Autodesk Inventor part; units mm, degrees
(part 2 of 2)
sketch "Sketch8" plane through (0, 0, 3) normal (0, 0, 1) x (1, 0, 0)
  line L0 (210.1, -2) -> (210.1, -24.3525) projected
  line L1 (210.1, -2) -> (212.6, -2)
  line L2 (212.6, -2) -> (212.6, -5)
  line L3 (212.6, -5) -> (210.1, -5)
  line L4 (210.1, -5) -> (210.1, -2)
  point P0 (0, 0)
  dimension "d104" = 2.5
  dimension "d105" = 3
  constraints: 8 end point, 2 parallel, 1 horizontal, 1 perpendicular
  measures "d104" distance of L2.end L3.end
  measures "d105" distance of L1.end L2.end
extrude "Extrusion8" cut sketch "Sketch8" against normal blind 2
equation "\"d1\" = d0"
equation "\"d2\" = sw"
equation "\"d3\" = sw"
equation "\"d4\" = sw"
equation "\"d5\" = sw"
equation "\"d6\" = sw"
equation "\"d7\" = sw"
equation "\"d8\" = sw"
equation "\"d9\" = sw"
equation "\"d10\" = sw"
equation "\"d11\" = sw"
equation "\"d12\" = sw"
equation "\"d13\" = sw"
equation "\"d14\" = sw"
equation "\"d15\" = sw"
equation "\"d16\" = sw"
equation "\"d17\" = sw"
equation "\"d18\" = sw"
equation "\"d19\" = sw"
equation "\"d20\" = sw"
equation "\"d21\" = sw"
equation "\"d22\" = sw"
equation "\"d23\" = sw"
equation "\"d24\" = sw"
equation "\"d25\" = sw"
equation "\"d26\" = sw"
equation "\"d27\" = sw"
equation "\"d30\" = sw"
equation "\"d31\" = sw"
equation "\"d32\" = sw"
equation "\"d33\" = sw"
equation "\"d34\" = sw"
equation "\"d35\" = sw"
equation "\"d36\" = sw"
equation "\"d37\" = sw"
equation "\"d38\" = sw"
equation "\"d39\" = sw"
equation "\"d40\" = sw"
equation "\"d41\" = sw"
equation "\"d42\" = sw"
equation "\"d43\" = sw"
equation "\"d44\" = sw"
equation "\"d45\" = sw"
equation "\"d46\" = sw"
equation "\"d47\" = sw"
equation "\"d48\" = sw"
equation "\"d49\" = sw"
equation "\"d50\" = sw"
equation "\"d51\" = sw"
equation "\"d52\" = sw"
equation "\"d53\" = sw"
equation "\"d55\" = sw"
equation "\"d56\" = sw"
equation "\"d58\" = d57"
equation "\"d64\" = d63"
equation "\"d66\" = d65"
equation "\"d67\" = d65"
equation "\"d68\" = d65"
equation "\"d69\" = d63"
equation "\"d71\" = d63"
equation "\"sw\" = 14.005"
body "Solid1"
